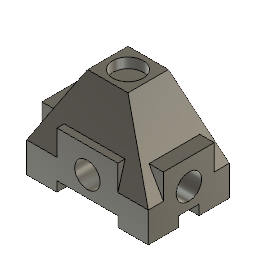
QWEQ (3) (Autodesk Fusion 360 design; units mm, degrees)
Autodesk Fusion 360 part; units mm, degrees
note: some values were not read from the file. Chosen so that the rebuilt part matches the saved one: that a step has no effect.
sketch "Sketch1" plane through (0, 0, 0) normal (0, 0, 1) x (1, 0, 0)
  line L0 (0, 10) -> (6, 10)
  line L1 (6, 10) -> (6, 14)
  line L2 (6, 14) -> (0, 14)
  line L3 (0, 14) -> (0, 10)
extrude "Extrude1" add sketch "Sketch1" along normal blind 1
move_body "Move1" bodies 1 to x (1, 0, 0) y (0, 1, 0) z (0, 0, 1) at (-3, 0, 0)
sketch "Sketch2" plane through (0, 0, 0) normal (1, 0, 0) x (0, 1, 0)
move_body "Move2" bodies 1 to x (1, 0, 0) y (0, 1, 0) z (0, 0, 1) at (0, 0, -4.5)
sketch "Sketch3" plane through (0, 0, 0) normal (1, 0, 0) x (0, 1, 0)
  line L0 (14, -3.5) -> (10, -3.5)
  line L1 (12, -3.5) -> (12, 0)
sketch "Sketch4" plane through (0, 0, 0) normal (0, 0, 1) x (1, 0, 0)
  line L0 (-1, 11) -> (1, 11)
  line L1 (1, 11) -> (1, 13)
  line L2 (1, 13) -> (-1, 13)
  line L3 (-1, 13) -> (-1, 11)
loft "Loft1" add profiles "Sketch4" section 1 face at (-1, 12.6667, -3.5) section 2
sketch "Sketch5" plane through (3, 0, 0) normal (1, 0, 0) x (0, 1, 0)
  line L0 (10, -4.5) -> (14, -4.5)
  line L1 (14, -4.5) -> (14, -3.5)
  line L2 (14, -3.5) -> (10, -3.5)
  line L3 (10, -3.5) -> (10, -4.5)
  line L4 (12, -3.5) -> (13.25, -3.5)
  line L5 (13.25, -3.5) -> (13.25, -2.25)
  line L6 (13.25, -2.25) -> (10.75, -2.25)
  line L7 (10.75, -2.25) -> (10.7456, -3.5)
  dimension "d3" = 1.25
  dimension "d4" = 2.5
form "Form1" [no effect]
extrude "Extrude2" cut sketch "Sketch5" against normal blind 6 contours L2 L4 L5 L6 L7
sketch "Sketch6" plane through (3, 0, 0) normal (1, 0, 0) x (0, 1, 0)
  line L0 (10, -4.5) -> (14, -4.5)
  line L1 (14, -4.5) -> (14, -3.5)
  line L2 (14, -3.5) -> (13.25, -3.5)
  line L3 (13.25, -3.5) -> (10.7456, -3.5)
  line L4 (10.7456, -3.5) -> (10, -3.5)
  line L5 (10, -3.5) -> (10, -4.5)
  line L6 (10.7456, -3.5) -> (13.25, -3.5)
  line L7 (13.25, -3.5) -> (13.25, -2.25)
  line L8 (13.25, -2.25) -> (10.7456, -2.25)
  line L9 (10.7456, -2.25) -> (10.7456, -3.5)
extrude "Extrude3" cut sketch "Sketch6" against normal blind 6 contours L3 L6 L7 L8 L9
sketch "Sketch7" plane through (-3, 0, 0) normal (-1, 0, 0) x (0, -1, 0)
  line L0 (-14, -4.5) -> (-10, -4.5)
  line L1 (-10, -4.5) -> (-10, -3.5)
  line L2 (-10, -3.5) -> (-10.7456, -3.5)
  line L3 (-10.7456, -3.5) -> (-13.25, -3.5)
  line L4 (-13.25, -3.5) -> (-14, -3.5)
  line L5 (-14, -3.5) -> (-14, -4.5)
  line L6 (-13.25, -3.5) -> (-10.7456, -3.5)
  line L7 (-10.7456, -3.5) -> (-10.7456, -2.25)
  line L8 (-10.7456, -2.25) -> (-13.25, -2.25)
  line L9 (-13.25, -2.25) -> (-13.25, -3.5)
extrude "Extrude4" add sketch "Sketch7" against normal blind 6 contours L3 L6 L7 L8 L9
sketch "Sketch8" plane through (0, 10, 0) normal (0, -1, 0) x (1, 0, 0)
  line L0 (-3, -4.5) -> (3, -4.5)
  line L1 (3, -4.5) -> (3, -3.5)
  line L2 (3, -3.5) -> (-3, -3.5)
  line L3 (-3, -3.5) -> (-3, -4.5)
  line L4 (0, -3.5) -> (-1.5, -3.5)
  line L5 (-1.5, -3.5) -> (1.5, -3.5)
  line L6 (1.5, -3.5) -> (1.5, -2.25)
  line L7 (1.5, -2.25) -> (-1.5, -2.25)
  line L8 (-1.5, -2.25) -> (-1.5, -3.5)
  dimension "d11" = 1.25
extrude "Extrude5" cut sketch "Sketch8" against normal blind 4 contours L2 L4 L5 L6 L7 L8
sketch "Sketch9" plane through (0, 14, 0) normal (0, 1, 0) x (-1, 0, 0)
  line L0 (-3, -4.5) -> (3, -4.5)
  line L1 (3, -4.5) -> (3, -3.5)
  line L2 (3, -3.5) -> (1.5, -3.5)
  line L3 (1.5, -3.5) -> (-1.5, -3.5)
  line L4 (-1.5, -3.5) -> (-3, -3.5)
  line L5 (-3, -3.5) -> (-3, -4.5)
  line L6 (-1.5, -3.5) -> (1.5, -3.5)
  line L7 (1.5, -3.5) -> (1.5, -2.25)
  line L8 (1.5, -2.25) -> (-1.5, -2.25)
  line L9 (-1.5, -2.25) -> (-1.5, -3.5)
extrude "Extrude6" add sketch "Sketch9" against normal blind 4 contours L3 L6 L7 L8 L9
sketch "Sketch18" plane through (0, 10, 0) normal (0, -1, 0) x (1, 0, 0)
  line L0 (-3, -4.5) -> (3, -4.5)
  line L1 (3, -4.5) -> (3, -3.5)
  line L2 (3, -3.5) -> (1.5, -3.5)
  line L3 (1.5, -3.5) -> (1.5, -2.25)
  line L4 (1.5, -2.25) -> (-1.5, -2.25)
  line L5 (-1.5, -2.25) -> (-1.5, -3.5)
  line L6 (-1.5, -3.5) -> (-3, -3.5)
  line L7 (-3, -3.5) -> (-3, -4.5)
  circle A0 centre (0, -3.5) radius 0.625
  dimension "d44" = 1.25
  measures "d44" diameter of A0
extrude "Extrude8" cut sketch "Sketch18" against normal blind 4 contours A0
sketch "Sketch19" plane through (-3, 0, 0) normal (-1, 0, 0) x (0, -1, 0)
  line L0 (-14, -4.5) -> (-10, -4.5)
  line L1 (-10, -4.5) -> (-10, -3.5)
  line L2 (-10, -3.5) -> (-10.7456, -3.5)
  line L3 (-10.7456, -3.5) -> (-10.7456, -2.25)
  line L4 (-10.7456, -2.25) -> (-13.25, -2.25)
  line L5 (-13.25, -2.25) -> (-13.25, -3.5)
  line L6 (-13.25, -3.5) -> (-14, -3.5)
  line L7 (-14, -3.5) -> (-14, -4.5)
  circle A0 centre (-12, -3.5) radius 0.625
  dimension "d47" = 1.25
  measures "d47" diameter of A0
extrude "Extrude9" cut sketch "Sketch19" against normal blind 6 contours A0
sketch "Sketch20" plane through (0, 0, 0) normal (0, 0, 1) x (-1, 0, 0)
  line L0 (-1, -13) -> (1, -13)
  line L1 (1, -13) -> (1, -11)
  line L2 (1, -11) -> (-1, -11)
  line L3 (-1, -11) -> (-1, -13)
  circle A0 centre (0, -12) radius 0.75
  dimension "d50" = 1.5
  measures "d50" diameter of A0
extrude "Extrude10" cut sketch "Sketch20" against normal blind 0.5 contours A0
sketch "Sketch21" plane through (0, 0, -4.5) normal (0, 0, -1) x (1, 0, 0)
  line L0 (-3, -10) -> (-3, -14)
  line L1 (-3, -14) -> (3, -14)
  line L2 (3, -14) -> (3, -10)
  line L3 (3, -10) -> (-3, -10)
  line L4 (-3, -14) -> (-1.5, -14)
  line L5 (-1.5, -14) -> (-1.5, -12.5)
  line L6 (-1.5, -12.5) -> (-3, -12.5)
  line L7 (-3, -12.5) -> (-3, -14)
extrude "Extrude11" add sketch "Sketch21" along normal blind 0.5 contours L0 L1 L4 L5 L6 L7
sketch "Sketch22" plane through (0, 0, -4.5) normal (0, 0, -1) x (1, 0, 0)
  line L0 (-1.5, -12.5) -> (-1.5, -14)
  line L1 (-1.5, -14) -> (3, -14)
  line L2 (3, -14) -> (3, -10)
  line L3 (3, -10) -> (-3, -10)
  line L4 (-3, -10) -> (-3, -12.5)
  line L5 (-3, -12.5) -> (-1.5, -12.5)
  line L6 (-3, -10) -> (-1.5, -10)
  line L7 (-1.5, -10) -> (-1.5, -11.5)
  line L8 (-1.5, -11.5) -> (-3, -11.5)
  line L9 (-3, -11.5) -> (-3, -10)
extrude "Extrude12" add sketch "Sketch22" along normal blind 1.5 contours L3 L4 L6 L7 L8 L9
extrude "Extrude13" cut 1 faces at (-2.5, 10.5, -6) along direction (0, 0, 1) blind 1
sketch "Sketch23" plane through (0, 0, -4.5) normal (0, 0, -1) x (1, 0, 0)
  line L0 (-1.5, -10) -> (-1.5, -11.5)
  line L1 (-1.5, -11.5) -> (-3, -11.5)
  line L2 (-3, -11.5) -> (-3, -12.5)
  line L3 (-3, -12.5) -> (-1.5, -12.5)
  line L4 (-1.5, -12.5) -> (-1.5, -14)
  line L5 (-1.5, -14) -> (3, -14)
  line L6 (3, -14) -> (3, -10)
  line L7 (3, -10) -> (-1.5, -10)
  line L8 (3, -10) -> (1.5, -10)
  line L9 (1.5, -10) -> (1.5, -11.5)
  line L10 (1.5, -11.5) -> (3, -11.5)
  line L11 (3, -11.5) -> (3, -10)
extrude "Extrude14" add sketch "Sketch23" along normal blind 0.5 contours L6 L7 L8 L9 L10 L11
sketch "Sketch24" plane through (0, 0, -4.5) normal (0, 0, -1) x (1, 0, 0)
  line L0 (1.5, -11.5) -> (1.5, -10)
  line L1 (1.5, -10) -> (-1.5, -10)
  line L2 (-1.5, -10) -> (-1.5, -11.5)
  line L3 (-1.5, -11.5) -> (-3, -11.5)
  line L4 (-3, -11.5) -> (-3, -12.5)
  line L5 (-3, -12.5) -> (-1.5, -12.5)
  line L6 (-1.5, -12.5) -> (-1.5, -14)
  line L7 (-1.5, -14) -> (3, -14)
  line L8 (3, -14) -> (3, -11.5)
  line L9 (3, -11.5) -> (1.5, -11.5)
  line L10 (3, -14) -> (1.5, -14)
  line L11 (1.5, -14) -> (1.5, -12.5)
  line L12 (1.5, -12.5) -> (3, -12.5)
  line L13 (3, -12.5) -> (3, -14)
extrude "Extrude15" add sketch "Sketch24" along normal blind 0.5 contours L7 L8 L10 L11 L12 L13
sketch "Sketch11" plane through (0, 14, 0) normal (0, 1, 0) x (-1, 0, 0)
  line L0 (-3, -4.5) -> (3, -4.5)
  line L1 (3, -4.5) -> (3, -3.5)
  line L2 (3, -3.5) -> (1.5, -3.5)
  line L3 (1.5, -3.5) -> (1.5, -2.25)
  line L4 (1.5, -2.25) -> (-1.5, -2.25)
  line L5 (-1.5, -2.25) -> (-1.5, -3.5)
  line L6 (-1.5, -3.5) -> (-3, -3.5)
  line L7 (-3, -3.5) -> (-3, -4.5)
  line L8 (-1.5, -3.5) -> (1.5, -3.5)
  line L9 (0, -2.25) -> (0, -4.5)
hole "Hole4" [rolled back] hole depth 1.375 hole diameter 1.25 tip angle 90
sketch "Sketch12" plane through (0, 10, 0) normal (0, -1, 0) x (1, 0, 0)
  line L0 (-3, -4.5) -> (3, -4.5)
  line L1 (3, -4.5) -> (3, -3.5)
  line L2 (3, -3.5) -> (1.5, -3.5)
  line L3 (1.5, -3.5) -> (1.5, -2.25)
  line L4 (1.5, -2.25) -> (-1.5, -2.25)
  line L5 (-1.5, -2.25) -> (-1.5, -3.5)
  line L6 (-1.5, -3.5) -> (-3, -3.5)
  line L7 (-3, -3.5) -> (-3, -4.5)
  line L8 (-1.5, -3.5) -> (1.5, -3.5)
  line L9 (0, -2.25) -> (0, -4.5)
  line L10 (0, -2.25) -> (0, -4.5)
hole "Hole7" [rolled back] hole depth 1.375 hole diameter 1.25 tip angle 90
hole "Hole5" [rolled back] hole depth 1.375 hole diameter 1.25 tip angle 90
sketch "Sketch14" plane through (-3, 0, 0) normal (-1, 0, 0) x (0, -1, 0)
  line L0 (-14, -4.5) -> (-10, -4.5)
  line L1 (-10, -4.5) -> (-10, -3.5)
  line L2 (-10, -3.5) -> (-10.7456, -3.5)
  line L3 (-10.7456, -3.5) -> (-10.7456, -2.25)
  line L4 (-10.7456, -2.25) -> (-13.25, -2.25)
  line L5 (-13.25, -2.25) -> (-13.25, -3.5)
  line L6 (-13.25, -3.5) -> (-14, -3.5)
  line L7 (-14, -3.5) -> (-14, -4.5)
sketch "Sketch15" plane through (3, 0, 0) normal (1, 0, 0) x (0, 1, 0)
  line L0 (10, -4.5) -> (14, -4.5)
  line L1 (14, -4.5) -> (14, -3.5)
  line L2 (14, -3.5) -> (13.25, -3.5)
  line L3 (13.25, -3.5) -> (13.25, -2.25)
  line L4 (13.25, -2.25) -> (10.7456, -2.25)
  line L5 (10.7456, -2.25) -> (10.7456, -3.5)
  line L6 (10.7456, -3.5) -> (10, -3.5)
  line L7 (10, -3.5) -> (10, -4.5)
  line L8 (10.7456, -3.5) -> (13.25, -3.5)
  line L9 (11.9978, -2.25) -> (12, -4.5)
hole "Hole8" [rolled back] hole depth 2.3738 hole diameter 1.25 tip angle 90
sketch "Sketch16" plane through (-3, 12.6239, -2.875) normal (-1, 0, 0) x (0, -1, 0)
  circle A0 centre (0.6252, -0.6251) radius 0.625
  dimension "d40" = 1.25
  measures "d40" diameter of A0
extrude "Extrude7" [rolled back] along distance -6 taper angle 0
sketch "Sketch17" plane through (0, 0, 0) normal (0, 0, 1) x (-1, 0, 0)
  line L0 (-1, -13) -> (1, -13)
  line L1 (1, -13) -> (1, -11)
  line L2 (1, -11) -> (-1, -11)
  line L3 (-1, -11) -> (-1, -13)
ref_plane "WorkPlane1" through (0, 12, 0) normal (0, 0, 1) x (-1, 0, 0)
sketch "Sketch13" plane through (3, 0, 0) normal (1, 0, 0) x (0, 1, 0)
  line L0 (10, -4.5) -> (14, -4.5)
  line L1 (14, -4.5) -> (14, -3.5)
  line L2 (14, -3.5) -> (13.25, -3.5)
  line L3 (13.25, -3.5) -> (13.25, -2.25)
  line L4 (13.25, -2.25) -> (10.7456, -2.25)
  line L5 (10.7456, -2.25) -> (10.7456, -3.5)
  line L6 (10.7456, -3.5) -> (10, -3.5)
  line L7 (10, -3.5) -> (10, -4.5)
  line L8 (10.7456, -3.5) -> (13.25, -3.5)
  line L9 (11.9978, -2.25) -> (12, -4.5)
hole "Hole6" [rolled back] hole depth 2.375 hole diameter 1.25 tip angle 90
hole "Hole1" [rolled back] hole depth 1.375 hole diameter 1.25 tip angle 90
hole "Hole2" [rolled back] hole depth 1.375 hole diameter 1.25 tip angle 90
sketch "Sketch10" plane through (-3, 0, 0) normal (-1, 0, 0) x (0, -1, 0)
  line L0 (-14, -4.5) -> (-10, -4.5)
  line L1 (-10, -4.5) -> (-10, -3.5)
  line L2 (-10, -3.5) -> (-10.7456, -3.5)
  line L3 (-10.7456, -3.5) -> (-10.7456, -2.25)
  line L4 (-10.7456, -2.25) -> (-13.25, -2.25)
  line L5 (-13.25, -2.25) -> (-13.25, -3.5)
  line L6 (-13.25, -3.5) -> (-14, -3.5)
  line L7 (-14, -3.5) -> (-14, -4.5)
  line L8 (-13.25, -3.5) -> (-10.7456, -3.5)
  line L9 (-11.9978, -2.25) -> (-11.9978, -4.5)
hole "Hole3" [rolled back] hole depth 2.375 hole diameter 1.25 tip angle 90
